Autodesk Fusion 360 part; units mm, degrees
(part 2 of 7)
sketch "草图4" plane through (0, 2, 0) normal (0, 1, 0) x (-1, 0, 0)
  spline S0 degree 3 poles (0.4584, 12.176) (0.7918, 12.3856) (1.2919, 12.7285) (1.5681, 12.9333) knots 0 0 0 0 1 1 1 1
  spline S1 degree 3 poles (1.5681, 12.9333) (2.0349, 13.2905) (2.4064, 13.5334) (2.4826, 13.5334) knots 0 0 0 0 1 1 1 1
  spline S2 degree 3 poles (2.4826, 13.5334) (2.5016, 13.5334) (2.5302, 13.5095) (2.5492, 13.4762) knots 0 0 0 0 1 1 1 1
  spline S3 degree 3 poles (2.5492, 13.4762) (2.5683, 13.4476) (2.5159, 13.3619) (2.4159, 13.2762) knots 0 0 0 0 1 1 1 1
  spline S4 degree 3 poles (2.4159, 13.2762) (2.2016, 13.0904) (1.3252, 12.4903) (1.0442, 12.3379) knots 0 0 0 0 1 1 1 1
  spline S5 degree 3 poles (1.0442, 12.3379) (0.9252, 12.276) (0.8014, 12.1951) (0.768, 12.1665) knots 0 0 0 0 1 1 1 1
  spline S6 degree 3 poles (0.768, 12.1665) (0.7347, 12.1331) (0.6728, 12.1046) (0.6299, 12.1046) knots 0 0 0 0 1 1 1 1
  spline S7 degree 3 poles (0.6299, 12.1046) (0.5918, 12.1046) (0.4775, 12.0331) (0.3775, 11.9474) knots 0 0 0 0 1 1 1 1
  spline S8 degree 3 poles (0.3775, 11.9474) (0.2727, 11.8617) (0.1298, 11.7569) (0.0584, 11.7188) knots 0 0 0 0 1 1 1 1
  spline S9 degree 3 poles (0.0584, 11.7188) (-0.0131, 11.6855) (-0.175, 11.5807) (-0.294, 11.4997) knots 0 0 0 0 1 1 1 1
  spline S10 degree 3 poles (-0.294, 11.4997) (-0.5417, 11.3235) (-0.637, 11.3045) (-0.6131, 11.4283) knots 0 0 0 0 1 1 1 1
  spline S11 degree 3 poles (-0.6131, 11.4283) (-0.5989, 11.514) (-0.5179, 11.5664) (0.4584, 12.176) knots 0 0 0 0 1 1 1 1
  spline S12 degree 3 poles (-2.9087, 11.6283) (-3.0564, 11.6283) (-3.0992, 11.6474) (-3.0992, 11.714) knots 0 0 0 0 1 1 1 1
  spline S13 degree 3 poles (-3.0992, 11.714) (-3.0992, 11.7855) (-3.0325, 11.795) (-2.5372, 11.8093) knots 0 0 0 0 1 1 1 1
  spline S14 degree 3 poles (-2.5372, 11.8093) (-2.2324, 11.8141) (-1.9324, 11.8093) (-1.8705, 11.795) knots 0 0 0 0 1 1 1 1
  spline S15 degree 3 poles (-1.8705, 11.795) (-1.68, 11.7474) (-1.7514, 11.6378) (-1.9895, 11.6045) knots 0 0 0 0 1 1 1 1
  spline S16 degree 3 poles (-1.9895, 11.6045) (-2.2229, 11.5712) (-2.4801, 11.4045) (-2.4801, 11.2806) knots 0 0 0 0 1 1 1 1
  spline S17 degree 3 poles (-2.4801, 11.2806) (-2.4801, 11.2473) (-2.4991, 11.1997) (-2.5229, 11.1759) knots 0 0 0 0 1 1 1 1
  spline S18 degree 3 poles (-2.5229, 11.1759) (-2.5468, 11.1473) (-2.7182, 10.7949) (-2.8992, 10.39) knots 0 0 0 0 1 1 1 1
  spline S19 degree 3 poles (-2.8992, 10.39) (-3.2373, 9.6423) (-3.8279, 8.4659) (-3.9184, 8.3516) knots 0 0 0 0 1 1 1 1
  spline S20 degree 3 poles (-3.9184, 8.3516) (-3.9946, 8.2659) (-4.0279, 8.3135) (-4.2137, 8.7803) knots 0 0 0 0 1 1 1 1
  spline S21 degree 3 poles (-4.2137, 8.7803) (-4.3042, 9.0089) (-4.4423, 9.3137) (-4.5185, 9.4661) knots 0 0 0 0 1 1 1 1
  line L0 (-4.5185, 9.4661) -> (-4.6566, 9.7376)
  line L1 (-4.6566, 9.7376) -> (-4.7947, 9.4089)
  spline S22 degree 3 poles (-4.7947, 9.4089) (-4.8709, 9.228) (-4.9471, 9.0755) (-4.9662, 9.066) knots 0 0 0 0 1 1 1 1
  spline S23 degree 3 poles (-4.9662, 9.066) (-4.99, 9.0565) (-5.0043, 9.0232) (-5.0043, 8.9898) knots 0 0 0 0 1 1 1 1
  spline S24 degree 3 poles (-5.0043, 8.9898) (-5.0043, 8.8946) (-5.2091, 8.4183) (-5.2662, 8.3802) knots 0 0 0 0 1 1 1 1
  spline S25 degree 3 poles (-5.2662, 8.3802) (-5.3424, 8.3278) (-5.4091, 8.4326) (-5.552, 8.8184) knots 0 0 0 0 1 1 1 1
  spline S26 degree 3 poles (-5.552, 8.8184) (-5.7091, 9.2375) (-6.0187, 9.9804) (-6.2616, 10.4996) knots 0 0 0 0 1 1 1 1
  spline S27 degree 3 poles (-6.2616, 10.4996) (-6.3569, 10.6996) (-6.4331, 10.8806) (-6.4331, 10.8949) knots 0 0 0 0 1 1 1 1
  spline S28 degree 3 poles (-6.4331, 10.8949) (-6.4331, 10.9758) (-6.695, 11.5188) (-6.7617, 11.5712) knots 0 0 0 0 1 1 1 1
  spline S29 degree 3 poles (-6.7617, 11.5712) (-6.7998, 11.5997) (-6.895, 11.6283) (-6.9712, 11.6283) knots 0 0 0 0 1 1 1 1
  spline S30 degree 3 poles (-6.9712, 11.6283) (-7.057, 11.6283) (-7.0998, 11.6474) (-7.0903, 11.6902) knots 0 0 0 0 1 1 1 1
  spline S31 degree 3 poles (-7.0903, 11.6902) (-7.076, 11.7283) (-6.9093, 11.7521) (-6.5331, 11.7617) knots 0 0 0 0 1 1 1 1
  spline S32 degree 3 poles (-6.5331, 11.7617) (-6.0425, 11.7712) (-5.9997, 11.7664) (-6.0139, 11.6902) knots 0 0 0 0 1 1 1 1
  spline S33 degree 3 poles (-6.0139, 11.6902) (-6.0235, 11.6378) (-6.0854, 11.595) (-6.1711, 11.5807) knots 0 0 0 0 1 1 1 1
  spline S34 degree 3 poles (-6.1711, 11.5807) (-6.2473, 11.5664) (-6.3045, 11.5426) (-6.2997, 11.5235) knots 0 0 0 0 1 1 1 1
  spline S35 degree 3 poles (-6.2997, 11.5235) (-6.2521, 11.3711) (-6.214, 11.2806) (-6.0901, 11.0092) knots 0 0 0 0 1 1 1 1
  spline S36 degree 3 poles (-6.0901, 11.0092) (-6.0092, 10.8377) (-5.8806, 10.552) (-5.8044, 10.3662) knots 0 0 0 0 1 1 1 1
  spline S37 degree 3 poles (-5.8044, 10.3662) (-5.7282, 10.1852) (-5.6377, 9.99) (-5.6044, 9.9376) knots 0 0 0 0 1 1 1 1
  spline S38 degree 3 poles (-5.6044, 9.9376) (-5.571, 9.8852) (-5.5043, 9.7376) (-5.4615, 9.6042) knots 0 0 0 0 1 1 1 1
  spline S39 degree 3 poles (-5.4615, 9.6042) (-5.4186, 9.4756) (-5.3519, 9.3137) (-5.3186, 9.2518) knots 0 0 0 0 1 1 1 1
  line L2 (-5.3186, 9.2518) -> (-5.2519, 9.1327)
  line L3 (-5.2519, 9.1327) -> (-5.1614, 9.3232)
  spline S40 degree 3 poles (-5.1614, 9.3232) (-5.109, 9.4232) (-5.0281, 9.609) (-4.9852, 9.728) knots 0 0 0 0 1 1 1 1
  spline S41 degree 3 poles (-4.9852, 9.728) (-4.9043, 9.9423) (-4.9043, 9.9566) (-5.0043, 10.2043) knots 0 0 0 0 1 1 1 1
  spline S42 degree 3 poles (-5.0043, 10.2043) (-5.1948, 10.6663) (-5.2519, 10.7901) (-5.3615, 11.0092) knots 0 0 0 0 1 1 1 1
  spline S43 degree 3 poles (-5.3615, 11.0092) (-5.4186, 11.1282) (-5.4853, 11.2902) (-5.4996, 11.3759) knots 0 0 0 0 1 1 1 1
  spline S44 degree 3 poles (-5.4996, 11.3759) (-5.5377, 11.5426) (-5.5996, 11.6093) (-5.7377, 11.6331) knots 0 0 0 0 1 1 1 1
  spline S45 degree 3 poles (-5.7377, 11.6331) (-5.7901, 11.6426) (-5.8377, 11.6807) (-5.852, 11.714) knots 0 0 0 0 1 1 1 1
  spline S46 degree 3 poles (-5.852, 11.714) (-5.8663, 11.7569) (-5.7425, 11.7712) (-5.3377, 11.7712) knots 0 0 0 0 1 1 1 1
  spline S47 degree 3 poles (-5.3377, 11.7712) (-4.8566, 11.7712) (-4.809, 11.7617) (-4.8233, 11.6902) knots 0 0 0 0 1 1 1 1
  spline S48 degree 3 poles (-4.8233, 11.6902) (-4.8328, 11.6378) (-4.8947, 11.595) (-4.9805, 11.5807) knots 0 0 0 0 1 1 1 1
  spline S49 degree 3 poles (-4.9805, 11.5807) (-5.0567, 11.5664) (-5.1281, 11.5235) (-5.1376, 11.4807) knots 0 0 0 0 1 1 1 1
  spline S50 degree 3 poles (-5.1376, 11.4807) (-5.1424, 11.4426) (-5.0757, 11.2425) (-4.9805, 11.0377) knots 0 0 0 0 1 1 1 1
  spline S51 degree 3 poles (-4.9805, 11.0377) (-4.89, 10.8377) (-4.8138, 10.6472) (-4.8138, 10.6186) knots 0 0 0 0 1 1 1 1
  spline S52 degree 3 poles (-4.8138, 10.6186) (-4.8138, 10.5281) (-4.6614, 10.2472) (-4.6233, 10.271) knots 0 0 0 0 1 1 1 1
  spline S53 degree 3 poles (-4.6233, 10.271) (-4.5566, 10.3091) (-4.3851, 10.7187) (-4.3851, 10.8282) knots 0 0 0 0 1 1 1 1
  spline S54 degree 3 poles (-4.3851, 10.8282) (-4.3899, 10.8901) (-4.428, 11.0235) (-4.4804, 11.1282) knots 0 0 0 0 1 1 1 1
  spline S55 degree 3 poles (-4.4804, 11.1282) (-4.5328, 11.233) (-4.5709, 11.3664) (-4.5756, 11.4283) knots 0 0 0 0 1 1 1 1
  spline S56 degree 3 poles (-4.5756, 11.4283) (-4.5756, 11.4854) (-4.609, 11.5473) (-4.6471, 11.5616) knots 0 0 0 0 1 1 1 1
  spline S57 degree 3 poles (-4.6471, 11.5616) (-4.6852, 11.5807) (-4.7185, 11.6331) (-4.7185, 11.6807) knots 0 0 0 0 1 1 1 1
  spline S58 degree 3 poles (-4.7185, 11.6807) (-4.7185, 11.7664) (-4.6757, 11.7712) (-4.1708, 11.7712) knots 0 0 0 0 1 1 1 1
  spline S59 degree 3 poles (-4.1708, 11.7712) (-3.6803, 11.7712) (-3.6231, 11.7617) (-3.6231, 11.6902) knots 0 0 0 0 1 1 1 1
  spline S60 degree 3 poles (-3.6231, 11.6902) (-3.6231, 11.6188) (-3.666, 11.6045) (-3.9041, 11.6045) knots 0 0 0 0 1 1 1 1
  spline S61 degree 3 poles (-3.9041, 11.6045) (-4.0613, 11.6045) (-4.2042, 11.5854) (-4.2232, 11.5664) knots 0 0 0 0 1 1 1 1
  spline S62 degree 3 poles (-4.2232, 11.5664) (-4.247, 11.5473) (-4.2327, 11.4616) (-4.1994, 11.3759) knots 0 0 0 0 1 1 1 1
  spline S63 degree 3 poles (-4.1994, 11.3759) (-4.1661, 11.2902) (-4.066, 11.033) (-3.9803, 10.7949) knots 0 0 0 0 1 1 1 1
  spline S64 degree 3 poles (-3.9803, 10.7949) (-3.8946, 10.5615) (-3.7565, 10.2186) (-3.6755, 10.0376) knots 0 0 0 0 1 1 1 1
  spline S65 degree 3 poles (-3.6755, 10.0376) (-3.5279, 9.7137) (-3.5231, 9.709) (-3.4517, 9.8138) knots 0 0 0 0 1 1 1 1
  spline S66 degree 3 poles (-3.4517, 9.8138) (-3.4088, 9.8709) (-3.2945, 10.1138) (-3.1945, 10.3567) knots 0 0 0 0 1 1 1 1
  spline S67 degree 3 poles (-3.1945, 10.3567) (-3.0945, 10.5996) (-2.9468, 10.9473) (-2.8659, 11.1282) knots 0 0 0 0 1 1 1 1
  spline S68 degree 3 poles (-2.8659, 11.1282) (-2.6658, 11.5807) (-2.6706, 11.6283) (-2.9087, 11.6283) knots 0 0 0 0 1 1 1 1
  spline S69 degree 3 poles (0.387, 11.6331) (0.2679, 11.6807) (0.2727, 11.6807) (0.5489, 11.8664) knots 0 0 0 0 1 1 1 1
  spline S70 degree 3 poles (0.5489, 11.8664) (0.7013, 11.9712) (0.8442, 12.0569) (0.868, 12.0569) knots 0 0 0 0 1 1 1 1
  spline S71 degree 3 poles (0.868, 12.0569) (0.8871, 12.0569) (0.9014, 11.6188) (0.9014, 11.0806) knots 0 0 0 0 1 1 1 1
  spline S72 degree 3 poles (0.9014, 11.0806) (0.9014, 10.5424) (0.9109, 10.1043) (0.9157, 10.1043) knots 0 0 0 0 1 1 1 1
  spline S73 degree 3 poles (0.9157, 10.1043) (0.9252, 10.1043) (1.049, 10.2186) (1.1919, 10.3567) knots 0 0 0 0 1 1 1 1
  spline S74 degree 3 poles (1.1919, 10.3567) (1.3348, 10.4948) (1.511, 10.6567) (1.5919, 10.7187) knots 0 0 0 0 1 1 1 1
  spline S75 degree 3 poles (1.5919, 10.7187) (1.7062, 10.8044) (1.7205, 10.833) (1.6634, 10.8711) knots 0 0 0 0 1 1 1 1
  spline S76 degree 3 poles (1.6634, 10.8711) (1.6253, 10.8949) (1.4967, 10.9092) (1.3776, 10.8996) knots 0 0 0 0 1 1 1 1
  spline S77 degree 3 poles (1.3776, 10.8996) (1.2157, 10.8949) (1.1633, 10.9092) (1.1633, 10.9615) knots 0 0 0 0 1 1 1 1
  spline S78 degree 3 poles (1.1633, 10.9615) (1.1633, 11.0187) (1.2633, 11.0377) (1.7015, 11.0473) knots 0 0 0 0 1 1 1 1
  spline S79 degree 3 poles (1.7015, 11.0473) (2.2349, 11.0616) (2.2397, 11.0568) (2.2254, 10.9568) knots 0 0 0 0 1 1 1 1
  spline S80 degree 3 poles (2.2254, 10.9568) (2.2158, 10.8853) (2.1349, 10.8091) (2.0063, 10.7425) knots 0 0 0 0 1 1 1 1
  spline S81 degree 3 poles (2.0063, 10.7425) (1.5919, 10.5234) (1.049, 10.009) (1.2347, 10.009) knots 0 0 0 0 1 1 1 1
  spline S82 degree 3 poles (1.2347, 10.009) (1.2633, 10.009) (1.2824, 9.9662) (1.2824, 9.9185) knots 0 0 0 0 1 1 1 1
  spline S83 degree 3 poles (1.2824, 9.9185) (1.2824, 9.8661) (1.3014, 9.8185) (1.3252, 9.809) knots 0 0 0 0 1 1 1 1
  spline S84 degree 3 poles (1.3252, 9.809) (1.3491, 9.8042) (1.4538, 9.6661) (1.5634, 9.5089) knots 0 0 0 0 1 1 1 1
  spline S85 degree 3 poles (1.5634, 9.5089) (1.8682, 9.0708) (2.0301, 8.9136) (2.1682, 8.9136) knots 0 0 0 0 1 1 1 1
  line L4 (2.1682, 8.9136) -> (2.292, 8.9136)
  line L5 (2.292, 8.9136) -> (2.1444, 9.0803)
  spline S86 degree 3 poles (2.1444, 9.0803) (2.0682, 9.1708) (1.9777, 9.3375) (1.9444, 9.447) knots 0 0 0 0 1 1 1 1
  spline S87 degree 3 poles (1.9444, 9.447) (1.8729, 9.7233) (1.9158, 10.1852) (2.0349, 10.4234) knots 0 0 0 0 1 1 1 1
  spline S88 degree 3 poles (2.0349, 10.4234) (2.1492, 10.6424) (2.6159, 11.0377) (2.8159, 11.0806) knots 0 0 0 0 1 1 1 1
  spline S89 degree 3 poles (2.8159, 11.0806) (3.1779, 11.1616) (3.6399, 10.8472) (3.8066, 10.4091) knots 0 0 0 0 1 1 1 1
  spline S90 degree 3 poles (3.8066, 10.4091) (3.8589, 10.2662) (3.9018, 10.1281) (3.9018, 10.1043) knots 0 0 0 0 1 1 1 1
  spline S91 degree 3 poles (3.9018, 10.1043) (3.9018, 10.0757) (3.5494, 10.0519) (3.0826, 10.0471) knots 0 0 0 0 1 1 1 1
  line L6 (3.0826, 10.0471) -> (2.2587, 10.0328)
  line L7 (2.2587, 10.0328) -> (2.2444, 9.8947)
  spline S92 degree 3 poles (2.2444, 9.8947) (2.2111, 9.628) (2.2825, 9.4423) (2.4826, 9.247) knots 0 0 0 0 1 1 1 1
  spline S93 degree 3 poles (2.4826, 9.247) (2.8493, 8.8993) (3.1207, 8.885) (3.5922, 9.1994) knots 0 0 0 0 1 1 1 1
  spline S94 degree 3 poles (3.5922, 9.1994) (3.9161, 9.4137) (3.9494, 9.4232) (3.9494, 9.3042) knots 0 0 0 0 1 1 1 1
  spline S95 degree 3 poles (3.9494, 9.3042) (3.9494, 9.1613) (3.6589, 8.8612) (3.4065, 8.7422) knots 0 0 0 0 1 1 1 1
  spline S96 degree 3 poles (3.4065, 8.7422) (3.1827, 8.6374) (3.1065, 8.6279) (2.3587, 8.6279) knots 0 0 0 0 1 1 1 1
  line L8 (2.3587, 8.6279) -> (1.5586, 8.6279)
  line L9 (1.5586, 8.6279) -> (1.5872, 8.7755)
  spline S97 degree 3 poles (1.5872, 8.7755) (1.611, 8.9041) (1.5777, 8.9755) (1.3252, 9.3089) knots 0 0 0 0 1 1 1 1
  spline S98 degree 3 poles (1.3252, 9.3089) (1.1633, 9.5232) (1.0252, 9.7233) (1.0109, 9.7566) knots 0 0 0 0 1 1 1 1
  spline S99 degree 3 poles (1.0109, 9.7566) (0.9442, 9.9281) (0.9014, 9.7709) (0.9014, 9.347) knots 0 0 0 0 1 1 1 1
  line L10 (0.9014, 9.347) -> (0.9014, 8.8708)
  line L11 (0.9014, 8.8708) -> (1.1062, 8.8565)
  spline S100 degree 3 poles (1.1062, 8.8565) (1.2681, 8.8469) (1.3062, 8.8231) (1.3062, 8.7469) knots 0 0 0 0 1 1 1 1
  spline S101 degree 3 poles (1.3062, 8.7469) (1.3062, 8.6517) (1.2729, 8.6517) (-0.4798, 8.6517) knots 0 0 0 0 1 1 1 1
  line L12 (-0.4798, 8.6517) -> (-2.2658, 8.6517)
  line L13 (-2.2658, 8.6517) -> (-2.2801, 8.7612)
  spline S102 degree 3 poles (-2.2801, 8.7612) (-2.2943, 8.866) (-2.2991, 8.866) (-2.4944, 8.7136) knots 0 0 0 0 1 1 1 1
  spline S103 degree 3 poles (-2.4944, 8.7136) (-2.6992, 8.5517) (-3.0611, 8.2516) (-3.5231, 7.8468) knots 0 0 0 0 1 1 1 1
  spline S104 degree 3 poles (-3.5231, 7.8468) (-3.6707, 7.7182) (-4.1851, 7.2229) (-4.6709, 6.7466) knots 0 0 0 0 1 1 1 1
  spline S105 degree 3 poles (-4.6709, 6.7466) (-5.5377, 5.8894) (-5.7663, 5.7131) (-5.7663, 5.9037) knots 0 0 0 0 1 1 1 1
  spline S106 degree 3 poles (-5.7663, 5.9037) (-5.7663, 5.956) (-5.5567, 6.1846) (-5.2519, 6.4704) knots 0 0 0 0 1 1 1 1
  spline S107 degree 3 poles (-5.2519, 6.4704) (-4.79, 6.9038) (-4.3661, 7.2753) (-2.742, 8.6993) knots 0 0 0 0 1 1 1 1
  spline S108 degree 3 poles (-2.742, 8.6993) (-2.442, 8.9612) (-2.0848, 9.3089) (-1.9467, 9.4708) knots 0 0 0 0 1 1 1 1
  spline S109 degree 3 poles (-1.9467, 9.4708) (-1.8086, 9.6328) (-1.4418, 10.0281) (-1.1323, 10.3567) knots 0 0 0 0 1 1 1 1
  spline S110 degree 3 poles (-1.1323, 10.3567) (-0.8275, 10.6805) (-0.575, 10.9711) (-0.575, 11.0044) knots 0 0 0 0 1 1 1 1
  spline S111 degree 3 poles (-0.575, 11.0044) (-0.575, 11.0377) (-0.7179, 11.0568) (-1.0132, 11.0568) knots 0 0 0 0 1 1 1 1
  spline S112 degree 3 poles (-1.0132, 11.0568) (-1.3513, 11.0568) (-1.4657, 11.0377) (-1.5371, 10.9758) knots 0 0 0 0 1 1 1 1
  spline S113 degree 3 poles (-1.5371, 10.9758) (-1.5847, 10.933) (-1.6704, 10.8758) (-1.7276, 10.8472) knots 0 0 0 0 1 1 1 1
  spline S114 degree 3 poles (-1.7276, 10.8472) (-1.7847, 10.8187) (-1.8752, 10.7044) (-1.9324, 10.5901) knots 0 0 0 0 1 1 1 1
  spline S115 degree 3 poles (-1.9324, 10.5901) (-2.0276, 10.3948) (-2.1467, 10.3186) (-2.1467, 10.4615) knots 0 0 0 0 1 1 1 1
  spline S116 degree 3 poles (-2.1467, 10.4615) (-2.1467, 10.4996) (-2.1229, 10.6329) (-2.0896, 10.7568) knots 0 0 0 0 1 1 1 1
  spline S117 degree 3 poles (-2.0896, 10.7568) (-2.061, 10.8853) (-2.0181, 11.0711) (-1.9943, 11.1711) knots 0 0 0 0 1 1 1 1
  line L14 (-1.9943, 11.1711) -> (-1.9467, 11.3568)
  line L15 (-1.9467, 11.3568) -> (-1.0465, 11.3283)
  spline S118 degree 3 poles (-1.0465, 11.3283) (-0.4988, 11.3092) (-0.1369, 11.3187) (-0.1226, 11.3473) knots 0 0 0 0 1 1 1 1
  spline S119 degree 3 poles (-0.1226, 11.3473) (-0.0893, 11.3997) (0.0012, 11.4045) (0.0822, 11.3473) knots 0 0 0 0 1 1 1 1
  spline S120 degree 3 poles (0.0822, 11.3473) (0.206, 11.2711) (0.0774, 11.0616) (-0.3464, 10.6424) knots 0 0 0 0 1 1 1 1
  spline S121 degree 3 poles (-0.3464, 10.6424) (-0.5798, 10.4138) (-1.0418, 9.9376) (-1.3704, 9.5899) knots 0 0 0 0 1 1 1 1
  line L16 (-1.3704, 9.5899) -> (-1.9705, 8.9612)
  line L17 (-1.9705, 8.9612) -> (-1.0227, 8.9708)
  line L18 (-1.0227, 8.9708) -> (-0.0797, 8.9851)
  line L19 (-0.0797, 8.9851) -> (-0.0369, 9.1756)
  spline S122 degree 3 poles (-0.0369, 9.1756) (0.0203, 9.4137) (0.025, 9.4185) (0.1155, 9.328) knots 0 0 0 0 1 1 1 1
  spline S123 degree 3 poles (0.1155, 9.328) (0.1584, 9.2851) (0.187, 9.1708) (0.187, 9.0565) knots 0 0 0 0 1 1 1 1
  spline S124 degree 3 poles (0.187, 9.0565) (0.187, 8.866) (0.1917, 8.8612) (0.3394, 8.8755) knots 0 0 0 0 1 1 1 1
  spline S125 degree 3 poles (0.3394, 8.8755) (0.4727, 8.8898) (0.4965, 8.9136) (0.5299, 9.0565) knots 0 0 0 0 1 1 1 1
  spline S126 degree 3 poles (0.5299, 9.0565) (0.5727, 9.247) (0.5775, 10.8377) (0.5346, 11.2854) knots 0 0 0 0 1 1 1 1
  spline S127 degree 3 poles (0.5346, 11.2854) (0.5108, 11.5521) (0.4965, 11.595) (0.387, 11.6331) knots 0 0 0 0 1 1 1 1
  spline S128 degree 3 poles (4.4876, 11.052) (4.6924, 11.0568) (4.7115, 11.0473) (4.7115, 10.9425) knots 0 0 0 0 1 1 1 1
  spline S129 degree 3 poles (4.7115, 10.9425) (4.7115, 10.7758) (4.7972, 10.7425) (4.9162, 10.8568) knots 0 0 0 0 1 1 1 1
  spline S130 degree 3 poles (4.9162, 10.8568) (5.183, 11.1044) (5.4973, 11.1663) (5.7878, 11.0282) knots 0 0 0 0 1 1 1 1
  spline S131 degree 3 poles (5.7878, 11.0282) (5.8783, 10.9854) (6.0164, 10.8711) (6.0926, 10.7758) knots 0 0 0 0 1 1 1 1
  line L20 (6.0926, 10.7758) -> (6.2355, 10.6043)
  line L21 (6.2355, 10.6043) -> (6.2403, 9.8423)
  spline S132 degree 3 poles (6.2403, 9.8423) (6.245, 8.9136) (6.2593, 8.8469) (6.4641, 8.8279) knots 0 0 0 0 1 1 1 1
  spline S133 degree 3 poles (6.4641, 8.8279) (6.5784, 8.8184) (6.6165, 8.7898) (6.6165, 8.7184) knots 0 0 0 0 1 1 1 1
  spline S134 degree 3 poles (6.6165, 8.7184) (6.6165, 8.6326) (6.5784, 8.6279) (6.045, 8.6279) knots 0 0 0 0 1 1 1 1
  spline S135 degree 3 poles (6.045, 8.6279) (5.7307, 8.6279) (5.4735, 8.6422) (5.4735, 8.666) knots 0 0 0 0 1 1 1 1
  spline S136 degree 3 poles (5.4735, 8.666) (5.4782, 8.7565) (5.5592, 8.8136) (5.7116, 8.8279) knots 0 0 0 0 1 1 1 1
  line L22 (5.7116, 8.8279) -> (5.8783, 8.8422)
  line L23 (5.8783, 8.8422) -> (5.8783, 9.6899)
  spline S137 degree 3 poles (5.8783, 9.6899) (5.8783, 10.4519) (5.8688, 10.5424) (5.7973, 10.5853) knots 0 0 0 0 1 1 1 1
  spline S138 degree 3 poles (5.7973, 10.5853) (5.7497, 10.6139) (5.7116, 10.6615) (5.7116, 10.6996) knots 0 0 0 0 1 1 1 1
  spline S139 degree 3 poles (5.7116, 10.6996) (5.7116, 10.7806) (5.4068, 10.8853) (5.2592, 10.8472) knots 0 0 0 0 1 1 1 1
  spline S140 degree 3 poles (5.2592, 10.8472) (5.202, 10.833) (5.0591, 10.7615) (4.9543, 10.6901) knots 0 0 0 0 1 1 1 1
  line L24 (4.9543, 10.6901) -> (4.7591, 10.5615)
  line L25 (4.7591, 10.5615) -> (4.7686, 9.7042)
  line L26 (4.7686, 9.7042) -> (4.7829, 8.8422)
  line L27 (4.7829, 8.8422) -> (4.9258, 8.8279)
  spline S141 degree 3 poles (4.9258, 8.8279) (5.0687, 8.8088) (5.1544, 8.7374) (5.1115, 8.666) knots 0 0 0 0 1 1 1 1
  spline S142 degree 3 poles (5.1115, 8.666) (5.0877, 8.6279) (3.9494, 8.6088) (3.9494, 8.6469) knots 0 0 0 0 1 1 1 1
  spline S143 degree 3 poles (3.9494, 8.6469) (3.9494, 8.7565) (4.0304, 8.8184) (4.1638, 8.8184) knots 0 0 0 0 1 1 1 1
  spline S144 degree 3 poles (4.1638, 8.8184) (4.2638, 8.8184) (4.3304, 8.8469) (4.3495, 8.8946) knots 0 0 0 0 1 1 1 1
  spline S145 degree 3 poles (4.3495, 8.8946) (4.3876, 8.9946) (4.3876, 10.4805) (4.3495, 10.671) knots 0 0 0 0 1 1 1 1
  spline S146 degree 3 poles (4.3495, 10.671) (4.3257, 10.7853) (4.2876, 10.8282) (4.178, 10.8568) knots 0 0 0 0 1 1 1 1
  spline S147 degree 3 poles (4.178, 10.8568) (3.8875, 10.9282) (4.0637, 11.0425) (4.4876, 11.052) knots 0 0 0 0 1 1 1 1
  circle A0 centre (0, 0) radius 14.0811
  spline S148 degree 3 poles (-5.2833, -10.8985) (-5.4134, -10.9708) (-5.5435, -11.0141) (-5.5724, -10.9925) knots 0 0 0 0 1 1 1 1
  spline S149 degree 3 poles (-5.5724, -10.9925) (-5.6013, -10.978) (-5.7024, -11.0069) (-5.8036, -11.0647) knots 0 0 0 0 1 1 1 1
  spline S150 degree 3 poles (-5.8036, -11.0647) (-6.0348, -11.1875) (-6.0348, -11.1875) (-5.9842, -11.0214) knots 0 0 0 0 1 1 1 1
  spline S151 degree 3 poles (-5.9842, -11.0214) (-5.9264, -10.8407) (-6.1359, -10.819) (-6.3527, -10.9852) knots 0 0 0 0 1 1 1 1
  spline S152 degree 3 poles (-6.3527, -10.9852) (-6.5333, -11.1225) (-7.0319, -11.1225) (-7.2342, -10.978) knots 0 0 0 0 1 1 1 1
  spline S153 degree 3 poles (-7.2342, -10.978) (-7.3859, -10.8769) (-7.3931, -10.819) (-7.3931, -9.8436) knots 0 0 0 0 1 1 1 1
  spline S154 degree 3 poles (-7.3931, -9.8436) (-7.3931, -9.0488) (-7.4148, -8.7815) (-7.5015, -8.6587) knots 0 0 0 0 1 1 1 1
  spline S155 degree 3 poles (-7.5015, -8.6587) (-7.5955, -8.5214) (-7.5955, -8.5069) (-7.4437, -8.4636) knots 0 0 0 0 1 1 1 1
  spline S156 degree 3 poles (-7.4437, -8.4636) (-7.227, -8.4058) (-6.7067, -8.4058) (-6.6489, -8.4708) knots 0 0 0 0 1 1 1 1
  spline S157 degree 3 poles (-6.6489, -8.4708) (-6.62, -8.4925) (-6.6851, -8.5936) (-6.7862, -8.6876) knots 0 0 0 0 1 1 1 1
  spline S158 degree 3 poles (-6.7862, -8.6876) (-6.9741, -8.861) (-6.9741, -8.8754) (-6.9452, -9.7208) knots 0 0 0 0 1 1 1 1
  spline S159 degree 3 poles (-6.9452, -9.7208) (-6.9235, -10.2844) (-6.8801, -10.6167) (-6.8223, -10.689) knots 0 0 0 0 1 1 1 1
  spline S160 degree 3 poles (-6.8223, -10.689) (-6.7212, -10.8118) (-6.4755, -10.8335) (-6.0998, -10.7612) knots 0 0 0 0 1 1 1 1
  line L28 (-6.0998, -10.7612) -> (-5.8758, -10.7179)
  line L29 (-5.8758, -10.7179) -> (-5.8758, -8.7093)
  line L30 (-5.8758, -8.7093) -> (-6.0781, -8.6225)
  line L31 (-6.0781, -8.6225) -> (-6.2732, -8.5431)
  line L32 (-6.2732, -8.5431) -> (-6.0565, -8.4853)
  spline S161 degree 3 poles (-6.0565, -8.4853) (-5.9408, -8.4491) (-5.6518, -8.4275) (-5.4206, -8.4347) knots 0 0 0 0 1 1 1 1
  line L33 (-5.4206, -8.4347) -> (-5.0016, -8.4419)
  line L34 (-5.0016, -8.4419) -> (-5.1894, -8.5936)
  spline S162 degree 3 poles (-5.1894, -8.5936) (-5.3773, -8.7454) (-5.3845, -8.7743) (-5.4206, -9.7352) knots 0 0 0 0 1 1 1 1
  line L35 (-5.4206, -9.7352) -> (-5.464, -10.7179)
  line L36 (-5.464, -10.7179) -> (-5.2544, -10.7468)
  line L37 (-5.2544, -10.7468) -> (-5.0449, -10.7685)
  line L38 (-5.0449, -10.7685) -> (-5.2833, -10.8985)
  spline S163 degree 3 poles (6.0388, -10.1399) (6.4289, -11.2742) (6.5662, -11.5271) (6.7541, -11.5271) knots 0 0 0 0 1 1 1 1
  spline S164 degree 3 poles (6.7541, -11.5271) (6.8624, -11.5271) (6.8624, -11.5416) (6.7685, -11.5994) knots 0 0 0 0 1 1 1 1
  spline S165 degree 3 poles (6.7685, -11.5994) (6.6312, -11.6861) (5.6341, -11.6933) (5.5836, -11.6066) knots 0 0 0 0 1 1 1 1
  spline S166 degree 3 poles (5.5836, -11.6066) (5.5619, -11.5705) (5.6052, -11.5271) (5.6847, -11.5055) knots 0 0 0 0 1 1 1 1
  spline S167 degree 3 poles (5.6847, -11.5055) (5.8003, -11.4766) (5.8292, -11.4043) (5.8292, -11.1948) knots 0 0 0 0 1 1 1 1
  spline S168 degree 3 poles (5.8292, -11.1948) (5.8292, -10.9347) (5.3018, -9.2439) (5.1862, -9.1211) knots 0 0 0 0 1 1 1 1
  spline S169 degree 3 poles (5.1862, -9.1211) (5.1067, -9.0416) (4.8321, -9.6341) (4.7382, -10.0893) knots 0 0 0 0 1 1 1 1
  spline S170 degree 3 poles (4.7382, -10.0893) (4.6154, -10.6673) (4.8683, -11.491) (5.1934, -11.5416) knots 0 0 0 0 1 1 1 1
  spline S171 degree 3 poles (5.1934, -11.5416) (5.3524, -11.5705) (5.3451, -11.5777) (5.1573, -11.6283) knots 0 0 0 0 1 1 1 1
  spline S172 degree 3 poles (5.1573, -11.6283) (5.0489, -11.6644) (4.6732, -11.6644) (4.3264, -11.6355) knots 0 0 0 0 1 1 1 1
  spline S173 degree 3 poles (4.3264, -11.6355) (3.8206, -11.5922) (3.7339, -11.5705) (3.8784, -11.5127) knots 0 0 0 0 1 1 1 1
  spline S174 degree 3 poles (3.8784, -11.5127) (4.2324, -11.3826) (4.3191, -11.2381) (4.2686, -10.8841) knots 0 0 0 0 1 1 1 1
  spline S175 degree 3 poles (4.2686, -10.8841) (4.218, -10.5373) (3.9362, -9.6919) (3.7556, -9.3306) knots 0 0 0 0 1 1 1 1
  line L39 (3.7556, -9.3306) -> (3.6472, -9.1283)
  line L40 (3.6472, -9.1283) -> (3.5316, -9.2945)
  spline S176 degree 3 poles (3.5316, -9.2945) (3.4738, -9.3812) (3.2498, -9.9014) (3.0475, -10.4361) knots 0 0 0 0 1 1 1 1
  spline S177 degree 3 poles (3.0475, -10.4361) (2.6356, -11.5127) (2.6356, -11.5055) (3.1559, -11.5344) knots 0 0 0 0 1 1 1 1
  spline S178 degree 3 poles (3.1559, -11.5344) (3.4015, -11.5416) (3.4015, -11.5488) (3.0836, -11.6066) knots 0 0 0 0 1 1 1 1
  spline S179 degree 3 poles (3.0836, -11.6066) (2.903, -11.6355) (2.5128, -11.6644) (2.2166, -11.6644) knots 0 0 0 0 1 1 1 1
  line L41 (2.2166, -11.6644) -> (1.6747, -11.6716)
  line L42 (1.6747, -11.6716) -> (1.9564, -11.5055)
  spline S180 degree 3 poles (1.9564, -11.5055) (2.2527, -11.332) (2.5056, -10.8913) (3.3004, -9.1283) knots 0 0 0 0 1 1 1 1
  spline S181 degree 3 poles (3.3004, -9.1283) (3.5099, -8.6587) (3.705, -8.2757) (3.7339, -8.2757) knots 0 0 0 0 1 1 1 1
  spline S182 degree 3 poles (3.7339, -8.2757) (3.7628, -8.2757) (3.9073, -8.5431) (4.0518, -8.8754) knots 0 0 0 0 1 1 1 1
  spline S183 degree 3 poles (4.0518, -8.8754) (4.5431, -9.9881) (4.5648, -10.0026) (4.7454, -9.4173) knots 0 0 0 0 1 1 1 1
  spline S184 degree 3 poles (4.7454, -9.4173) (4.9116, -8.9043) (5.1862, -8.2757) (5.2512, -8.2757) knots 0 0 0 0 1 1 1 1
  spline S185 degree 3 poles (5.2512, -8.2757) (5.3307, -8.2757) (5.6414, -9.0055) (6.0388, -10.1399) knots 0 0 0 0 1 1 1 1
  spline S186 degree 3 poles (-3.1735, -8.6587) (-2.6244, -9.085) (-2.4366, -10.0459) (-2.8267, -10.4795) knots 0 0 0 0 1 1 1 1
  spline S187 degree 3 poles (-2.8267, -10.4795) (-3.123, -10.819) (-3.3108, -10.9563) (-3.6143, -11.0647) knots 0 0 0 0 1 1 1 1
  spline S188 degree 3 poles (-3.6143, -11.0647) (-3.9539, -11.1803) (-4.055, -11.1875) (-4.3657, -11.0864) knots 0 0 0 0 1 1 1 1
  spline S189 degree 3 poles (-4.3657, -11.0864) (-4.6692, -10.9852) (-4.9365, -10.7468) (-4.9365, -10.5878) knots 0 0 0 0 1 1 1 1
  spline S190 degree 3 poles (-4.9365, -10.5878) (-4.9365, -10.3422) (-4.6764, -10.2121) (-4.055, -10.1471) knots 0 0 0 0 1 1 1 1
  spline S191 degree 3 poles (-4.055, -10.1471) (-3.0218, -10.0315) (-3.0363, -10.0387) (-3.0868, -9.7208) knots 0 0 0 0 1 1 1 1
  spline S192 degree 3 poles (-3.0868, -9.7208) (-3.1952, -9.0127) (-3.4264, -8.8176) (-4.1128, -8.8249) knots 0 0 0 0 1 1 1 1
  spline S193 degree 3 poles (-4.1128, -8.8249) (-4.4308, -8.8249) (-4.6331, -8.8754) (-4.8209, -8.9838) knots 0 0 0 0 1 1 1 1
  spline S194 degree 3 poles (-4.8209, -8.9838) (-5.1388, -9.1717) (-5.1605, -9.085) (-4.8643, -8.796) knots 0 0 0 0 1 1 1 1
  spline S195 degree 3 poles (-4.8643, -8.796) (-4.4308, -8.3624) (-3.6504, -8.2974) (-3.1735, -8.6587) knots 0 0 0 0 1 1 1 1
  spline S196 degree 3 poles (1.9131, -10.4578) (1.9564, -10.978) (1.8914, -11.0141) (0.8943, -11.043) knots 0 0 0 0 1 1 1 1
  spline S197 degree 3 poles (0.8943, -11.043) (0.4102, -11.0503) (-0.0594, -11.0719) (-0.1461, -11.0792) knots 0 0 0 0 1 1 1 1
  spline S198 degree 3 poles (-0.1461, -11.0792) (-0.2328, -11.0864) (-0.3195, -11.0647) (-0.3484, -11.0286) knots 0 0 0 0 1 1 1 1
  spline S199 degree 3 poles (-0.3484, -11.0286) (-0.3701, -10.9925) (-0.0667, -10.5589) (0.3235, -10.0676) knots 0 0 0 0 1 1 1 1
  spline S200 degree 3 poles (0.3235, -10.0676) (0.7137, -9.5763) (1.1255, -9.0561) (1.2339, -8.9116) knots 0 0 0 0 1 1 1 1
  line L43 (1.2339, -8.9116) -> (1.4362, -8.637)
  line L44 (1.4362, -8.637) -> (0.8654, -8.637)
  spline S201 degree 3 poles (0.8654, -8.637) (0.2151, -8.637) (0.0562, -8.7165) (-0.1678, -9.1283) knots 0 0 0 0 1 1 1 1
  spline S202 degree 3 poles (-0.1678, -9.1283) (-0.2906, -9.374) (-0.3051, -9.3812) (-0.3123, -9.215) knots 0 0 0 0 1 1 1 1
  spline S203 degree 3 poles (-0.3123, -9.215) (-0.3123, -9.1139) (-0.2545, -8.8971) (-0.1895, -8.7309) knots 0 0 0 0 1 1 1 1
  line L45 (-0.1895, -8.7309) -> (-0.0594, -8.4202)
  line L46 (-0.0594, -8.4202) -> (1.075, -8.4202)
  spline S204 degree 3 poles (1.075, -8.4202) (1.8914, -8.4202) (2.2166, -8.4419) (2.2166, -8.5069) knots 0 0 0 0 1 1 1 1
  spline S205 degree 3 poles (2.2166, -8.5069) (2.2166, -8.6153) (1.7469, -9.215) (1.0027, -10.0676) knots 0 0 0 0 1 1 1 1
  spline S206 degree 3 poles (1.0027, -10.0676) (0.3163, -10.8552) (0.3235, -10.8985) (1.0894, -10.8263) knots 0 0 0 0 1 1 1 1
  spline S207 degree 3 poles (1.0894, -10.8263) (1.5663, -10.7829) (1.5735, -10.7757) (1.7325, -10.4867) knots 0 0 0 0 1 1 1 1
  line L47 (1.7325, -10.4867) -> (1.8914, -10.1904)
  line L48 (1.8914, -10.1904) -> (1.9131, -10.4578)
  spline S208 degree 3 poles (-0.4279, -11.7078) (-0.1245, -11.7945) (-0.1389, -11.8378) (-0.4929, -11.9173) knots 0 0 0 0 1 1 1 1
  spline S209 degree 3 poles (-0.4929, -11.9173) (-0.7675, -11.9896) (-0.8903, -12.0907) (-0.8903, -12.2569) knots 0 0 0 0 1 1 1 1
  spline S210 degree 3 poles (-0.8903, -12.2569) (-0.8903, -12.4086) (-1.071, -12.4447) (-1.1505, -12.3075) knots 0 0 0 0 1 1 1 1
  spline S211 degree 3 poles (-1.1505, -12.3075) (-1.1794, -12.2641) (-1.1938, -11.6572) (-1.1866, -10.9708) knots 0 0 0 0 1 1 1 1
  line L49 (-1.1866, -10.9708) -> (-1.1721, -9.7136)
  line L50 (-1.1721, -9.7136) -> (-1.3455, -9.8292)
  spline S212 degree 3 poles (-1.3455, -9.8292) (-1.4395, -9.887) (-1.6707, -10.1326) (-1.8513, -10.3711) knots 0 0 0 0 1 1 1 1
  line L51 (-1.8513, -10.3711) -> (-2.1837, -10.7974)
  line L52 (-2.1837, -10.7974) -> (-1.9236, -10.819)
  spline S213 degree 3 poles (-1.9236, -10.819) (-1.7791, -10.8335) (-1.649, -10.8841) (-1.6273, -10.9347) knots 0 0 0 0 1 1 1 1
  spline S214 degree 3 poles (-1.6273, -10.9347) (-1.6056, -10.9997) (-1.7502, -11.0214) (-2.1837, -11.0214) knots 0 0 0 0 1 1 1 1
  spline S215 degree 3 poles (-2.1837, -11.0214) (-2.5088, -11.0214) (-2.7689, -10.9925) (-2.7689, -10.9563) knots 0 0 0 0 1 1 1 1
  spline S216 degree 3 poles (-2.7689, -10.9563) (-2.7689, -10.9202) (-2.5883, -10.7323) (-2.3715, -10.5517) knots 0 0 0 0 1 1 1 1
  spline S217 degree 3 poles (-2.3715, -10.5517) (-2.1548, -10.3639) (-1.9958, -10.1832) (-2.0175, -10.1471) knots 0 0 0 0 1 1 1 1
  spline S218 degree 3 poles (-2.0175, -10.1471) (-2.0392, -10.111) (-2.0175, -10.0893) (-1.9669, -10.0965) knots 0 0 0 0 1 1 1 1
  spline S219 degree 3 poles (-1.9669, -10.0965) (-1.9163, -10.111) (-1.8296, -10.0315) (-1.7646, -9.9231) knots 0 0 0 0 1 1 1 1
  spline S220 degree 3 poles (-1.7646, -9.9231) (-1.649, -9.728) (-1.649, -9.7208) (-2.1186, -9.2439) knots 0 0 0 0 1 1 1 1
  spline S221 degree 3 poles (-2.1186, -9.2439) (-2.3788, -8.9838) (-2.7183, -8.702) (-2.8773, -8.6153) knots 0 0 0 0 1 1 1 1
  line L53 (-2.8773, -8.6153) -> (-3.1663, -8.4564)
  line L54 (-3.1663, -8.4564) -> (-2.5955, -8.4347)
  spline S222 degree 3 poles (-2.5955, -8.4347) (-1.9814, -8.413) (-1.9091, -8.4347) (-2.0392, -8.5936) knots 0 0 0 0 1 1 1 1
  spline S223 degree 3 poles (-2.0392, -8.5936) (-2.1042, -8.6731) (-2.0319, -8.7743) (-1.6707, -9.1283) knots 0 0 0 0 1 1 1 1
  line L55 (-1.6707, -9.1283) -> (-1.2155, -9.5691)
  line L56 (-1.2155, -9.5691) -> (-1.1721, -9.3306)
  spline S224 degree 3 poles (-1.1721, -9.3306) (-1.0999, -8.8899) (-1.1721, -8.5936) (-1.3817, -8.5142) knots 0 0 0 0 1 1 1 1
  spline S225 degree 3 poles (-1.3817, -8.5142) (-1.5478, -8.4491) (-1.4756, -8.4347) (-0.9843, -8.4275) knots 0 0 0 0 1 1 1 1
  spline S226 degree 3 poles (-0.9843, -8.4275) (-0.399, -8.4202) (-0.1967, -8.4997) (-0.5652, -8.5936) knots 0 0 0 0 1 1 1 1
  line L57 (-0.5652, -8.5936) -> (-0.7458, -8.637)
  line L58 (-0.7458, -8.637) -> (-0.7314, -10.1326)
  line L59 (-0.7314, -10.1326) -> (-0.7097, -11.6283)
  line L60 (-0.7097, -11.6283) -> (-0.4279, -11.7078)
  line L61 (-8.1905, -18.2474) -> (3.4998, -18.2474)
  line L62 (3.4998, -18.2474) -> (3.4998, -0.712)
  line L63 (3.4998, -0.712) -> (3.4998, 16.8234)
  line L64 (3.4998, 16.8234) -> (-8.1905, 16.8234)
  line L65 (-8.1905, 16.8234) -> (-19.8808, 16.8234)
  line L66 (-19.8808, 16.8234) -> (-19.8808, -0.712)
  line L67 (-19.8808, -0.712) -> (-19.8808, -18.2474)
  line L68 (-19.8808, -18.2474) -> (-8.1905, -18.2474)
  spline S227 degree 3 poles (-12.3643, -1.4517) (-12.2912, -1.3467) (-12.1451, -1.3193) (-12.0949, -1.3969) knots 0 0 0 0 1 1 1 1
  spline S228 degree 3 poles (-12.0949, -1.3969) (-12.0812, -1.4198) (-12.0994, -1.4883) (-12.136, -1.5431) knots 0 0 0 0 1 1 1 1
  spline S229 degree 3 poles (-12.136, -1.5431) (-12.2456, -1.6983) (-12.2227, -1.8764) (-12.0766, -2.05) knots 0 0 0 0 1 1 1 1
  spline S230 degree 3 poles (-12.0766, -2.05) (-11.8802, -2.2692) (-11.5834, -2.4153) (-10.8391, -2.6436) knots 0 0 0 0 1 1 1 1
  spline S231 degree 3 poles (-10.8391, -2.6436) (-10.1861, -2.8491) (-6.8434, -3.6939) (-6.4644, -3.7533) knots 0 0 0 0 1 1 1 1
  spline S232 degree 3 poles (-6.4644, -3.7533) (-6.3593, -3.7715) (-6.2589, -3.7989) (-6.2497, -3.8172) knots 0 0 0 0 1 1 1 1
  spline S233 degree 3 poles (-6.2497, -3.8172) (-6.1949, -3.904) (-6.5831, -3.9862) (-8.4371, -4.2739) knots 0 0 0 0 1 1 1 1
  spline S234 degree 3 poles (-8.4371, -4.2739) (-8.9074, -4.3469) (-9.3047, -4.4154) (-9.3139, -4.4245) knots 0 0 0 0 1 1 1 1
  spline S235 degree 3 poles (-9.3139, -4.4245) (-9.3321, -4.4428) (-8.6746, -4.6026) (-7.6654, -4.8218) knots 0 0 0 0 1 1 1 1
  spline S236 degree 3 poles (-7.6654, -4.8218) (-7.3411, -4.8949) (-7.0215, -4.9725) (-6.9575, -4.9954) knots 0 0 0 0 1 1 1 1
  line L69 (-6.9575, -4.9954) -> (-6.8434, -5.041)
  line L70 (-6.8434, -5.041) -> (-6.9575, -5.0684)
  spline S237 degree 3 poles (-6.9575, -5.0684) (-7.0215, -5.0821) (-7.3274, -5.1461) (-7.6425, -5.21) knots 0 0 0 0 1 1 1 1
  spline S238 degree 3 poles (-7.6425, -5.21) (-8.3275, -5.3515) (-9.3504, -5.6027) (-9.8801, -5.7671) knots 0 0 0 0 1 1 1 1
  spline S239 degree 3 poles (-9.8801, -5.7671) (-10.8162, -6.0457) (-11.2592, -6.4338) (-11.2592, -6.9681) knots 0 0 0 0 1 1 1 1
  spline S240 degree 3 poles (-11.2592, -6.9681) (-11.2546, -7.475) (-10.8893, -7.7992) (-10.5697, -7.58) knots 0 0 0 0 1 1 1 1
  spline S241 degree 3 poles (-10.5697, -7.58) (-10.4098, -7.4658) (-10.3459, -7.5709) (-10.5012, -7.6942) knots 0 0 0 0 1 1 1 1
  spline S242 degree 3 poles (-10.5012, -7.6942) (-10.7477, -7.886) (-11.1176, -7.7672) (-11.2729, -7.443) knots 0 0 0 0 1 1 1 1
  spline S243 degree 3 poles (-11.2729, -7.443) (-11.3916, -7.1964) (-11.4145, -6.7124) (-11.3231, -6.4338) knots 0 0 0 0 1 1 1 1
  spline S244 degree 3 poles (-11.3231, -6.4338) (-11.0994, -5.7625) (-10.5377, -5.4657) (-8.8526, -5.1415) knots 0 0 0 0 1 1 1 1
  spline S245 degree 3 poles (-8.8526, -5.1415) (-8.5787, -5.0913) (-8.3001, -5.0319) (-8.2362, -5.0182) knots 0 0 0 0 1 1 1 1
  line L71 (-8.2362, -5.0182) -> (-8.122, -4.9954)
  line L72 (-8.122, -4.9954) -> (-8.2362, -4.9497)
  spline S246 degree 3 poles (-8.2362, -4.9497) (-8.428, -4.8766) (-9.9166, -4.4565) (-10.3322, -4.3606) knots 0 0 0 0 1 1 1 1
  spline S247 degree 3 poles (-10.3322, -4.3606) (-11.0628, -4.1917) (-11.0583, -4.1643) (-10.2591, -4.1232) knots 0 0 0 0 1 1 1 1
  spline S248 degree 3 poles (-10.2591, -4.1232) (-9.9395, -4.1049) (-9.2545, -4.0318) (-8.7385, -3.9542) knots 0 0 0 0 1 1 1 1
  spline S249 degree 3 poles (-8.7385, -3.9542) (-8.2225, -3.8811) (-7.711, -3.8172) (-7.5969, -3.8172) knots 0 0 0 0 1 1 1 1
  spline S250 degree 3 poles (-7.5969, -3.8172) (-7.4781, -3.8172) (-7.4142, -3.7989) (-7.437, -3.7761) knots 0 0 0 0 1 1 1 1
  spline S251 degree 3 poles (-7.437, -3.7761) (-7.5512, -3.6711) (-8.6974, -3.3697) (-9.9714, -3.1094) knots 0 0 0 0 1 1 1 1
  spline S252 degree 3 poles (-9.9714, -3.1094) (-11.1724, -2.8628) (-11.3597, -2.8171) (-11.6565, -2.6756) knots 0 0 0 0 1 1 1 1
  spline S253 degree 3 poles (-11.6565, -2.6756) (-11.9487, -2.534) (-12.2775, -2.2326) (-12.3734, -2.0134) knots 0 0 0 0 1 1 1 1
  spline S254 degree 3 poles (-12.3734, -2.0134) (-12.4556, -1.8262) (-12.4511, -1.575) (-12.3643, -1.4517) knots 0 0 0 0 1 1 1 1
  spline S255 degree 3 poles (-11.6839, 2.3019) (-11.5971, 2.4663) (-11.4464, 2.5896) (-11.3642, 2.5622) knots 0 0 0 0 1 1 1 1
  spline S256 degree 3 poles (-11.3642, 2.5622) (-11.2775, 2.5257) (-11.2775, 2.4207) (-11.3597, 2.3476) knots 0 0 0 0 1 1 1 1
  spline S257 degree 3 poles (-11.3597, 2.3476) (-11.3962, 2.3202) (-11.4601, 2.206) (-11.5012, 2.101) knots 0 0 0 0 1 1 1 1
  spline S258 degree 3 poles (-11.5012, 2.101) (-11.5606, 1.9549) (-11.5652, 1.8818) (-11.5241, 1.7813) knots 0 0 0 0 1 1 1 1
  spline S259 degree 3 poles (-11.5241, 1.7813) (-11.3551, 1.3293) (-9.7568, 0.2607) (-8.8526, -0.0087) knots 0 0 0 0 1 1 1 1
  spline S260 degree 3 poles (-8.8526, -0.0087) (-8.3229, -0.164) (-8.2362, -0.1823) (-8.2362, -0.1412) knots 0 0 0 0 1 1 1 1
  spline S261 degree 3 poles (-8.2362, -0.1412) (-8.2362, -0.0955) (-8.5695, 0.3475) (-8.775, 0.5758) knots 0 0 0 0 1 1 1 1
  spline S262 degree 3 poles (-8.775, 0.5758) (-8.8846, 0.6945) (-8.9714, 0.7493) (-9.0581, 0.7493) knots 0 0 0 0 1 1 1 1
  spline S263 degree 3 poles (-9.0581, 0.7493) (-9.2225, 0.7493) (-9.3687, 0.9091) (-9.3047, 1.0142) knots 0 0 0 0 1 1 1 1
  spline S264 degree 3 poles (-9.3047, 1.0142) (-9.2773, 1.0553) (-9.1997, 1.0964) (-9.1312, 1.1055) knots 0 0 0 0 1 1 1 1
  spline S265 degree 3 poles (-9.1312, 1.1055) (-9.0307, 1.1192) (-8.9577, 1.0644) (-8.7294, 0.8178) knots 0 0 0 0 1 1 1 1
  spline S266 degree 3 poles (-8.7294, 0.8178) (-8.4051, 0.4708) (-8.3092, 0.3292) (-8.2316, 0.0735) knots 0 0 0 0 1 1 1 1
  spline S267 degree 3 poles (-8.2316, 0.0735) (-8.1768, -0.1183) (-8.1311, -0.1457) (-7.5284, -0.3786) knots 0 0 0 0 1 1 1 1
  spline S268 degree 3 poles (-7.5284, -0.3786) (-7.3183, -0.4562) (-7.3, -0.4745) (-7.3137, -0.5978) knots 0 0 0 0 1 1 1 1
  spline S269 degree 3 poles (-7.3137, -0.5978) (-7.3366, -0.7713) (-7.332, -0.7668) (-7.4781, -0.712) knots 0 0 0 0 1 1 1 1
  spline S270 degree 3 poles (-7.4781, -0.712) (-7.5466, -0.6891) (-7.8937, -0.6024) (-8.2499, -0.5247) knots 0 0 0 0 1 1 1 1
  spline S271 degree 3 poles (-8.2499, -0.5247) (-8.9348, -0.374) (-9.2773, -0.2416) (-9.9851, 0.1602) knots 0 0 0 0 1 1 1 1
  spline S272 degree 3 poles (-9.9851, 0.1602) (-10.7249, 0.5804) (-11.2318, 0.9959) (-11.5286, 1.4252) knots 0 0 0 0 1 1 1 1
  spline S273 degree 3 poles (-11.5286, 1.4252) (-11.7843, 1.7905) (-11.8254, 2.0188) (-11.6839, 2.3019) knots 0 0 0 0 1 1 1 1
  spline S274 degree 3 poles (-9.2088, 3.8408) (-9.0901, 3.9185) (-8.6883, 3.9093) (-8.0763, 3.8089) knots 0 0 0 0 1 1 1 1
  spline S275 degree 3 poles (-8.0763, 3.8089) (-7.4233, 3.7038) (-7.0945, 3.7632) (-7.0352, 3.9915) knots 0 0 0 0 1 1 1 1
  spline S276 degree 3 poles (-7.0352, 3.9915) (-7.0169, 4.0692) (-7.0534, 4.1057) (-7.2361, 4.197) knots 0 0 0 0 1 1 1 1
  spline S277 degree 3 poles (-7.2361, 4.197) (-7.3594, 4.261) (-7.4599, 4.334) (-7.4599, 4.3569) knots 0 0 0 0 1 1 1 1
  spline S278 degree 3 poles (-7.4599, 4.3569) (-7.4599, 4.4893) (-6.9119, 4.2975) (-6.8251, 4.1377) knots 0 0 0 0 1 1 1 1
  spline S279 degree 3 poles (-6.8251, 4.1377) (-6.6973, 3.9002) (-6.816, 3.6125) (-7.1082, 3.4618) knots 0 0 0 0 1 1 1 1
  spline S280 degree 3 poles (-7.1082, 3.4618) (-7.332, 3.3477) (-7.8617, 3.334) (-8.4188, 3.4344) knots 0 0 0 0 1 1 1 1
  spline S281 degree 3 poles (-8.4188, 3.4344) (-8.9759, 3.5349) (-9.0855, 3.5212) (-8.9029, 3.3751) knots 0 0 0 0 1 1 1 1
  spline S282 degree 3 poles (-8.9029, 3.3751) (-8.6974, 3.2107) (-7.9576, 2.859) (-7.6562, 2.7768) knots 0 0 0 0 1 1 1 1
  spline S283 degree 3 poles (-7.6562, 2.7768) (-7.3868, 2.7038) (-7.3685, 2.6946) (-7.3685, 2.5668) knots 0 0 0 0 1 1 1 1
  spline S284 degree 3 poles (-7.3685, 2.5668) (-7.3685, 2.4024) (-7.437, 2.375) (-7.7384, 2.4298) knots 0 0 0 0 1 1 1 1
  spline S285 degree 3 poles (-7.7384, 2.4298) (-7.8754, 2.4572) (-7.9896, 2.4709) (-7.9987, 2.4663) knots 0 0 0 0 1 1 1 1
  spline S286 degree 3 poles (-7.9987, 2.4663) (-8.0033, 2.4572) (-7.8937, 2.3659) (-7.7521, 2.2563) knots 0 0 0 0 1 1 1 1
  spline S287 degree 3 poles (-7.7521, 2.2563) (-7.469, 2.0416) (-7.2315, 1.7083) (-7.2315, 1.5211) knots 0 0 0 0 1 1 1 1
  spline S288 degree 3 poles (-7.2315, 1.5211) (-7.2315, 1.4571) (-7.2818, 1.3247) (-7.3457, 1.2334) knots 0 0 0 0 1 1 1 1
  line L73 (-7.3457, 1.2334) -> (-7.4553, 1.069)
  line L74 (-7.4553, 1.069) -> (-7.2726, 1.069)
  spline S289 degree 3 poles (-7.2726, 1.069) (-7.0671, 1.069) (-6.7566, 0.9274) (-6.711, 0.8178) knots 0 0 0 0 1 1 1 1
  spline S290 degree 3 poles (-6.711, 0.8178) (-6.6425, 0.6351) (-6.6836, 0.4662) (-6.8342, 0.3155) knots 0 0 0 0 1 1 1 1
  spline S291 degree 3 poles (-6.8342, 0.3155) (-7.0078, 0.142) (-7.1996, 0.0826) (-7.7019, 0.0506) knots 0 0 0 0 1 1 1 1
  spline S292 degree 3 poles (-7.7019, 0.0506) (-7.9804, 0.0324) (-8.0672, 0.0415) (-8.1266, 0.0963) knots 0 0 0 0 1 1 1 1
  spline S293 degree 3 poles (-8.1266, 0.0963) (-8.1905, 0.1602) (-8.1859, 0.1785) (-8.0946, 0.2744) knots 0 0 0 0 1 1 1 1
  line L75 (-8.0946, 0.2744) -> (-7.9941, 0.384)
  line L76 (-7.9941, 0.384) -> (-8.1129, 0.384)
  spline S294 degree 3 poles (-8.1129, 0.384) (-8.2088, 0.384) (-8.2362, 0.4068) (-8.2362, 0.4799) knots 0 0 0 0 1 1 1 1
  spline S295 degree 3 poles (-8.2362, 0.4799) (-8.2362, 0.6078) (-8.1585, 0.7356) (-8.0489, 0.7995) knots 0 0 0 0 1 1 1 1
  spline S296 degree 3 poles (-8.0489, 0.7995) (-7.8571, 0.9) (-7.6836, 0.5941) (-7.8663, 0.4662) knots 0 0 0 0 1 1 1 1
  spline S297 degree 3 poles (-7.8663, 0.4662) (-7.9393, 0.416) (-7.9028, 0.4068) (-7.5969, 0.3931) knots 0 0 0 0 1 1 1 1
  spline S298 degree 3 poles (-7.5969, 0.3931) (-7.2955, 0.384) (-7.2315, 0.3931) (-7.1219, 0.4799) knots 0 0 0 0 1 1 1 1
  spline S299 degree 3 poles (-7.1219, 0.4799) (-6.9301, 0.6306) (-6.9712, 0.7904) (-7.2544, 0.9411) knots 0 0 0 0 1 1 1 1
  spline S300 degree 3 poles (-7.2544, 0.9411) (-7.4507, 1.0507) (-7.5284, 1.069) (-7.8297, 1.0598) knots 0 0 0 0 1 1 1 1
  spline S301 degree 3 poles (-7.8297, 1.0598) (-8.1494, 1.0553) (-8.1996, 1.0644) (-8.4234, 1.2014) knots 0 0 0 0 1 1 1 1
  spline S302 degree 3 poles (-8.4234, 1.2014) (-8.8481, 1.4617) (-9.0444, 1.6489) (-9.1266, 1.8681) knots 0 0 0 0 1 1 1 1
  spline S303 degree 3 poles (-9.1266, 1.8681) (-9.2043, 2.0645) (-9.2043, 2.0736) (-9.0992, 2.2882) knots 0 0 0 0 1 1 1 1
  spline S304 degree 3 poles (-9.0992, 2.2882) (-8.9759, 2.5348) (-8.8389, 2.5896) (-8.6837, 2.4526) knots 0 0 0 0 1 1 1 1
  spline S305 degree 3 poles (-8.6837, 2.4526) (-8.5467, 2.3339) (-8.2362, 1.8453) (-8.2362, 1.7539) knots 0 0 0 0 1 1 1 1
  spline S306 degree 3 poles (-8.2362, 1.7539) (-8.2362, 1.5804) (-8.0855, 1.4754) (-7.7932, 1.4389) knots 0 0 0 0 1 1 1 1
  spline S307 degree 3 poles (-7.7932, 1.4389) (-7.4553, 1.3978) (-7.3685, 1.4389) (-7.3685, 1.6215) knots 0 0 0 0 1 1 1 1
  spline S308 degree 3 poles (-7.3685, 1.6215) (-7.3685, 1.7311) (-7.4325, 1.8224) (-7.7019, 2.0782) knots 0 0 0 0 1 1 1 1
  spline S309 degree 3 poles (-7.7019, 2.0782) (-7.88, 2.2563) (-8.0809, 2.4252) (-8.1448, 2.4572) knots 0 0 0 0 1 1 1 1
  spline S310 degree 3 poles (-8.1448, 2.4572) (-8.2773, 2.5257) (-8.9714, 2.7038) (-9.1723, 2.722) knots 0 0 0 0 1 1 1 1
  spline S311 degree 3 poles (-9.1723, 2.722) (-9.2773, 2.7312) (-9.3139, 2.7631) (-9.323, 2.8408) knots 0 0 0 0 1 1 1 1
  spline S312 degree 3 poles (-9.323, 2.8408) (-9.3504, 3.0326) (-9.2728, 3.0737) (-9.0033, 3.0052) knots 0 0 0 0 1 1 1 1
  spline S313 degree 3 poles (-9.0033, 3.0052) (-8.8709, 2.9686) (-8.6928, 2.9412) (-8.6015, 2.9412) knots 0 0 0 0 1 1 1 1
  spline S314 degree 3 poles (-8.6015, 2.9412) (-8.4462, 2.9412) (-8.4554, 2.9504) (-8.8298, 3.1696) knots 0 0 0 0 1 1 1 1
  spline S315 degree 3 poles (-8.8298, 3.1696) (-9.0444, 3.2929) (-9.2499, 3.439) (-9.2956, 3.4892) knots 0 0 0 0 1 1 1 1
  spline S316 degree 3 poles (-9.2956, 3.4892) (-9.3869, 3.6034) (-9.355, 3.7449) (-9.2088, 3.8408) knots 0 0 0 0 1 1 1 1
  spline S317 degree 3 poles (-9.1221, -0.6161) (-9.0079, -0.5065) (-9.0033, -0.5065) (-8.9394, -0.5978) knots 0 0 0 0 1 1 1 1
  spline S318 degree 3 poles (-8.9394, -0.5978) (-8.7522, -0.849) (-8.3686, -1.2645) (-8.1083, -1.4883) knots 0 0 0 0 1 1 1 1
  spline S319 degree 3 poles (-8.1083, -1.4883) (-7.7613, -1.7851) (-7.1311, -2.2646) (-7.0854, -2.2646) knots 0 0 0 0 1 1 1 1
  spline S320 degree 3 poles (-7.0854, -2.2646) (-7.0306, -2.2646) (-7.0397, -1.8125) (-7.0945, -1.6161) knots 0 0 0 0 1 1 1 1
  spline S321 degree 3 poles (-7.0945, -1.6161) (-7.1265, -1.5065) (-7.2087, -1.3969) (-7.3229, -1.3056) knots 0 0 0 0 1 1 1 1
  spline S322 degree 3 poles (-7.3229, -1.3056) (-7.4233, -1.2234) (-7.5055, -1.1412) (-7.5055, -1.1184) knots 0 0 0 0 1 1 1 1
  spline S323 degree 3 poles (-7.5055, -1.1184) (-7.5055, -1.0956) (-7.3685, -1.0773) (-7.1996, -1.0773) knots 0 0 0 0 1 1 1 1
  line L77 (-7.1996, -1.0773) -> (-6.889, -1.0773)
  line L78 (-6.889, -1.0773) -> (-6.8799, -1.7257)
  spline S324 degree 3 poles (-6.8799, -1.7257) (-6.8662, -2.4929) (-6.7977, -2.7532) (-6.5694, -2.9313) knots 0 0 0 0 1 1 1 1
  spline S325 degree 3 poles (-6.5694, -2.9313) (-6.4872, -2.9952) (-6.3411, -3.0592) (-6.2497, -3.0729) knots 0 0 0 0 1 1 1 1
  spline S326 degree 3 poles (-6.2497, -3.0729) (-5.9483, -3.1231) (-5.994, -3.3149) (-6.3091, -3.3149) knots 0 0 0 0 1 1 1 1
  spline S327 degree 3 poles (-6.3091, -3.3149) (-6.4278, -3.3149) (-6.5192, -3.2555) (-6.8114, -2.9815) knots 0 0 0 0 1 1 1 1
  spline S328 degree 3 poles (-6.8114, -2.9815) (-7.0032, -2.7989) (-7.3366, -2.5066) (-7.5512, -2.3331) knots 0 0 0 0 1 1 1 1
  spline S329 degree 3 poles (-7.5512, -2.3331) (-7.7658, -2.1596) (-8.1174, -1.8582) (-8.3366, -1.6572) knots 0 0 0 0 1 1 1 1
  spline S330 degree 3 poles (-8.3366, -1.6572) (-8.5558, -1.4609) (-8.7568, -1.3056) (-8.7796, -1.3148) knots 0 0 0 0 1 1 1 1
  spline S331 degree 3 poles (-8.7796, -1.3148) (-8.8481, -1.3376) (-8.4417, -2.3285) (-8.3092, -2.4609) knots 0 0 0 0 1 1 1 1
  spline S332 degree 3 poles (-8.3092, -2.4609) (-8.1631, -2.6071) (-8.1631, -2.6482) (-8.3001, -2.7349) knots 0 0 0 0 1 1 1 1
  spline S333 degree 3 poles (-8.3001, -2.7349) (-8.3869, -2.7943) (-8.4417, -2.7989) (-8.5741, -2.7623) knots 0 0 0 0 1 1 1 1
  spline S334 degree 3 poles (-8.5741, -2.7623) (-8.7933, -2.703) (-8.807, -2.6619) (-8.6654, -2.4975) knots 0 0 0 0 1 1 1 1
  spline S335 degree 3 poles (-8.6654, -2.4975) (-8.5513, -2.3605) (-8.5513, -2.3468) (-8.6152, -2.2052) knots 0 0 0 0 1 1 1 1
  spline S336 degree 3 poles (-8.6152, -2.2052) (-9.0216, -1.3467) (-9.2362, -0.849) (-9.2408, -0.7759) knots 0 0 0 0 1 1 1 1
  spline S337 degree 3 poles (-9.2408, -0.7759) (-9.2408, -0.7485) (-9.186, -0.68) (-9.1221, -0.6161) knots 0 0 0 0 1 1 1 1
  spline S338 degree 3 poles (-8.0535, 6.5396) (-7.8754, 6.9963) (-7.7293, 7.2109) (-7.5055, 7.3251) knots 0 0 0 0 1 1 1 1
  spline S339 degree 3 poles (-7.5055, 7.3251) (-7.0626, 7.5488) (-6.7292, 7.3662) (-6.5466, 6.7999) knots 0 0 0 0 1 1 1 1
  spline S340 degree 3 poles (-6.5466, 6.7999) (-6.4507, 6.494) (-6.4415, 6.3753) (-6.405, 4.2884) knots 0 0 0 0 1 1 1 1
  spline S341 degree 3 poles (-6.405, 4.2884) (-6.3776, 2.4207) (-6.3, 0.8863) (-6.2041, 0.1557) knots 0 0 0 0 1 1 1 1
  spline S342 degree 3 poles (-6.2041, 0.1557) (-5.9392, -1.8125) (-5.6926, -3.1094) (-5.2862, -4.6163) knots 0 0 0 0 1 1 1 1
  spline S343 degree 3 poles (-5.2862, -4.6163) (-5.1446, -5.1415) (-5.0122, -5.6118) (-4.9848, -5.6575) knots 0 0 0 0 1 1 1 1
  spline S344 degree 3 poles (-4.9848, -5.6575) (-4.962, -5.7032) (-4.9528, -5.7534) (-4.962, -5.7671) knots 0 0 0 0 1 1 1 1
  spline S345 degree 3 poles (-4.962, -5.7671) (-5.0122, -5.8173) (-5.4095, -4.8264) (-5.6515, -4.0455) knots 0 0 0 0 1 1 1 1
  spline S346 degree 3 poles (-5.6515, -4.0455) (-5.8387, -3.4336) (-6.236, -1.4928) (-6.3411, -0.6663) knots 0 0 0 0 1 1 1 1
  spline S347 degree 3 poles (-6.3411, -0.6663) (-6.542, 0.9685) (-6.5603, 1.2379) (-6.5877, 4.0372) knots 0 0 0 0 1 1 1 1
  line L79 (-6.5877, 4.0372) -> (-6.6151, 6.7999)
  line L80 (-6.6151, 6.7999) -> (-6.7292, 7.0054)
  spline S348 degree 3 poles (-6.7292, 7.0054) (-7.0352, 7.5534) (-7.4553, 7.3479) (-7.7795, 6.494) knots 0 0 0 0 1 1 1 1
  spline S349 degree 3 poles (-7.7795, 6.494) (-7.9211, 6.1241) (-8.0078, 6.0008) (-8.1311, 6.0008) knots 0 0 0 0 1 1 1 1
  spline S350 degree 3 poles (-8.1311, 6.0008) (-8.2225, 6.0008) (-8.2042, 6.1561) (-8.0535, 6.5396) knots 0 0 0 0 1 1 1 1
  spline S351 degree 3 poles (-8.8663, 1.8087) (-8.7294, 1.7265) (-8.3914, 1.5713) (-8.3412, 1.5713) knots 0 0 0 0 1 1 1 1
  spline S352 degree 3 poles (-8.3412, 1.5713) (-8.3321, 1.5713) (-8.3275, 1.6489) (-8.3366, 1.7402) knots 0 0 0 0 1 1 1 1
  spline S353 degree 3 poles (-8.3366, 1.7402) (-8.3458, 1.8772) (-8.3823, 1.932) (-8.533, 2.0371) knots 0 0 0 0 1 1 1 1
  spline S354 degree 3 poles (-8.533, 2.0371) (-8.6335, 2.1056) (-8.7841, 2.1786) (-8.8663, 2.1923) knots 0 0 0 0 1 1 1 1
  spline S355 degree 3 poles (-8.8663, 2.1923) (-9.0079, 2.2197) (-9.0125, 2.2197) (-9.0125, 2.0599) knots 0 0 0 0 1 1 1 1
  spline S356 degree 3 poles (-9.0125, 2.0599) (-9.0125, 1.9275) (-8.9851, 1.8818) (-8.8663, 1.8087) knots 0 0 0 0 1 1 1 1
  line L81 (8.273, 16.9407) -> (-2.9614, 16.9407)
  line L82 (-2.9614, 16.9407) -> (-2.9614, 0.0891)
  line L83 (-2.9614, 0.0891) -> (-2.9614, -16.7625)
  line L84 (-2.9614, -16.7625) -> (8.273, -16.7625)
  line L85 (8.273, -16.7625) -> (19.5074, -16.7625)
  line L86 (19.5074, -16.7625) -> (19.5074, 0.0891)
  line L87 (19.5074, 0.0891) -> (19.5074, 16.9407)
  line L88 (19.5074, 16.9407) -> (8.273, 16.9407)
  spline S357 degree 3 poles (11.6214, -1.2889) (11.4064, -1.1309) (11.1782, -0.9422) (11.1036, -0.8764) knots 0 0 0 0 1 1 1 1
  spline S358 degree 3 poles (11.1036, -0.8764) (11.0334, -0.8106) (10.8842, -0.7008) (10.7832, -0.6394) knots 0 0 0 0 1 1 1 1
  line L89 (10.7832, -0.6394) -> (10.5901, -0.5209)
  line L90 (10.5901, -0.5209) -> (9.5983, -0.5253)
  spline S359 degree 3 poles (9.5983, -0.5253) (9.0542, -0.5253) (8.5978, -0.5385) (8.589, -0.5473) knots 0 0 0 0 1 1 1 1
  spline S360 degree 3 poles (8.589, -0.5473) (8.5583, -0.578) (8.6855, -0.7579) (8.984, -1.1046) knots 0 0 0 0 1 1 1 1
  line L91 (8.984, -1.1046) -> (9.256, -1.4162)
  line L92 (9.256, -1.4162) -> (9.3175, -1.2318)
  spline S361 degree 3 poles (9.3175, -1.2318) (9.3658, -1.0826) (9.3921, -1.0563) (9.4404, -1.1002) knots 0 0 0 0 1 1 1 1
  spline S362 degree 3 poles (9.4404, -1.1002) (9.4842, -1.1353) (9.5018, -1.2626) (9.5018, -1.5566) knots 0 0 0 0 1 1 1 1